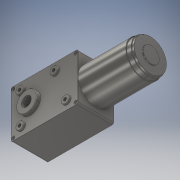
# Autodesk Inventor part: TS-58GZ868D
Saved by Autodesk Inventor 2018 (Build 220112000, 112)
## iProperties
Created: 2018-04-10
Part Number: TS-58GZ868D
Material: Steel, Cast
Document SubType Name: Modeling
Designer: P136265
Density: 7.85 g/cm^3
Appearance: Semi-Polished
Author: P136265
Autodesk Inventor part; units mm, degrees
ref_plane "YZ Plane" through (0, 0, 0) normal (1, 0, 0) x (0, 1, 0)
ref_plane "XZ Plane" through (0, 0, 0) normal (0, 1, 0) x (-1, 0, 0)
ref_plane "XY Plane" through (0, 0, 0) normal (0, 0, 1) x (1, 0, 0)
sketch "Sketch1" plane through (0, 0, 0) normal (0, 1, 0) x (-1, 0, 0)
  line L0 (-39.25, 29) -> (39.25, 29)
  line L1 (41.25, 27) -> (41.25, -27)
  line L2 (39.25, -29) -> (-39.25, -29)
  line L3 (-41.25, -27) -> (-41.25, 27)
  line L4 (-41.25, 29) -> (41.25, -29) construction
  line L5 (41.25, 29) -> (-41.25, -29) construction
  arc A0 (41.25, 27) -> (39.25, 29) centre (39.25, 27) ccw
  arc A1 (-39.25, 29) -> (-41.25, 27) centre (-39.25, 27) ccw
  arc A2 (-41.25, -27) -> (-39.25, -29) centre (-39.25, -27) ccw
  arc A3 (39.25, -29) -> (41.25, -27) centre (39.25, -27) ccw
  point P0 (0, 0)
  dimension "d0" = 82.5
  dimension "d1" = 58
  dimension "d2" = 2
  constraints: 12 end point, 8 point on circle, 8 point on line, 8 tangent, 4 centre point, 3 equal radius, 2 midpoint, 2 parallel, 1 horizontal, 1 perpendicular
  measures "d0" distance of L4.end L5.end
  measures "d1" distance of L5.start L4.end
  measures "d2" radius of A0
extrude "Extrusion1" add sketch "Sketch1" along normal mid plane 44
sketch "Sketch2" plane through (0, 22, 0) normal (0, 1, 0) x (1, 0, 0)
  line L0 (-41.25, 27) -> (-41.25, -27) construction
  arc A0 (-41.25, -27) -> (-39.25, -29) centre (-39.25, -27) ccw construction
  line L1 (-39.25, -29) -> (39.25, -29) construction
  arc A1 (39.25, -29) -> (41.25, -27) centre (39.25, -27) ccw construction
  line L2 (41.25, -27) -> (41.25, 27) construction
  arc A2 (41.25, 27) -> (39.25, 29) centre (39.25, 27) ccw construction
  line L3 (39.25, 29) -> (-39.25, 29) construction
  arc A3 (-39.25, 29) -> (-41.25, 27) centre (-39.25, 27) ccw construction
  line L4 (39.25, -29) -> (-39.25, -29) construction
  line L5 (28.25, -29) -> (28.25, 29) construction
  line L6 (-39.25, 29) -> (39.25, 29) construction
  line L7 (17.25, -29) -> (17.25, 29) construction
  circle A4 centre (17.25, 0) radius 12.5
  point P0 (0, 0)
  dimension "d5" = 13
  dimension "d7" = 11
  dimension "d8" = 25
  constraints: 4 end point, 4 point on line, 2 perpendicular, 1 centre point, 1 midpoint
  measures "d5" distance between parallel lines of L2 L5
  measures "d7" distance between parallel lines of L5 L7
  measures "d8" diameter of A4
extrude "Extrusion2" add sketch "Sketch2" along normal blind 5
sketch "Sketch3" plane through (0, 22, 0) normal (0, 1, 0) x (1, 0, 0)
  circle A0 centre (17.25, 0) radius 12.5 construction
  line L0 (-41.25, 27) -> (-41.25, -27) construction
  arc A1 (-41.25, -27) -> (-39.25, -29) centre (-39.25, -27) ccw construction
  line L1 (-39.25, -29) -> (39.25, -29) construction
  arc A2 (39.25, -29) -> (41.25, -27) centre (39.25, -27) ccw construction
  line L2 (41.25, -27) -> (41.25, 27) construction
  arc A3 (41.25, 27) -> (39.25, 29) centre (39.25, 27) ccw construction
  line L3 (39.25, 29) -> (-39.25, 29) construction
  arc A4 (-39.25, 29) -> (-41.25, 27) centre (-39.25, 27) ccw construction
  line L4 (28.25, -29) -> (28.25, 29) construction
  circle A5 centre (28.25, -19) radius 5
  circle A6 centre (28.25, 19) radius 5
  line L5 (28.25, 0) -> (17.25, 0) construction
  line L6 (-39.25, -29) -> (39.25, -29) construction
  line L7 (17.25, -29) -> (17.25, 29) construction
  line L8 (-13.75, -29) -> (-13.75, 29) construction
  line L9 (-27.75, -29) -> (-27.75, 29) construction
  circle A7 centre (-13.75, -19) radius 5
  circle A8 centre (-27.75, 19) radius 5
  line L10 (17.25, 0) -> (-27.75, 0) construction
  point P0 (0, 0)
  dimension "d11" = 13
  dimension "d12" = 10
  dimension "d13" = 10
  dimension "d14" = 38
  dimension "d15" = 19
  dimension "d19" = 31
  dimension "d20" = 45
  dimension "d21" = 10
  dimension "d22" = 10
  dimension "d23" = 19
  dimension "d24" = 19
  constraints: 12 end point, 12 point on line, 4 centre point, 4 perpendicular, 3 midpoint, 1 horizontal
  measures "d11" distance between parallel lines of L2 L4
  measures "d12" diameter of A5
  measures "d13" diameter of A6
  measures "d14" distance of A6.centre A5.centre
  measures "d15" distance of L5.start A5.centre
  measures "d19" distance from line of L5.end L8
  measures "d20" distance between parallel lines of L9 L7
  measures "d21" diameter of A7
  measures "d22" diameter of A8
  measures "d23" distance from line of L10 A8.centre
  measures "d24" distance from line of L10 A7.centre
extrude "Extrusion3" add sketch "Sketch3" along normal blind 2.5
fillet "Fillet1" radius 0.5 5 edges at (-18.75, 24.5, 19) (-32.75, 24.5, -19) (23.25, 24.5, 19) (23.25, 24.5, -19) (4.75, 27, 0)
mirror "Mirror1" about plane through (0, 0, 0) normal (0, 1, 0) of "Extrusion3", "Extrusion2", "Fillet1"
sketch "Sketch6" plane through (-13.75, 24.5, 19) normal (0, 1, 0) x (1, 0, 0)
  circle A0 centre (0, 0) radius 4.5 construction
  circle A1 centre (-14, 38) radius 4.5 construction
  circle A2 centre (42, 38) radius 4.5 construction
  circle A3 centre (42, 0) radius 4.5 construction
  point P0 (13.75, 19)
hole "Hole1" at (-13.75, 24.5, 19) at (-27.75, 24.5, -19) at (28.25, 24.5, -19) at (28.25, 24.5, 19) direction (0, -1, 0) diameter 4 end through all
thread "Thread1" size "M4x0.7" class "6H" standard "ANSI Metric M Profile" full length
thread "Thread2" size "M4x0.7" class "6H" standard "ANSI Metric M Profile" full length
thread "Thread3" size "M4x0.7" class "6H" standard "ANSI Metric M Profile" full length
thread "Thread4" size "M4x0.7" class "6H" standard "ANSI Metric M Profile" full length
sketch "Sketch7" plane through (-41.25, -22, 27) normal (-1, 0, 0) x (0, 0, 1)
  circle A0 centre (-27, 22) radius 22
  dimension "d51" = 44
  constraints: 1 centre point, 1 coincident
  measures "d51" diameter of A0
extrude "Extrusion6" add sketch "Sketch7" along normal blind 59
sketch "Sketch8" plane through (-100.25, 0, 0) normal (-1, 0, 0) x (0, 0, 1)
  circle A0 centre (0, 0) radius 21
  dimension "d54" = 42
  constraints: 1 centre point, 1 coincident
  measures "d54" diameter of A0
extrude "Extrusion7" add sketch "Sketch8" along normal blind 5.5
sketch "Sketch9" plane through (-105.75, 0, 0) normal (-1, 0, 0) x (0, 0, 1)
  circle A0 centre (0, 0) radius 20
  dimension "d57" = 40
  constraints: 1 centre point, 1 coincident
  measures "d57" diameter of A0
extrude "Extrusion8" add sketch "Sketch9" along normal blind 2.5
sketch "Sketch10" plane through (-108.25, 0, 0) normal (-1, 0, 0) x (0, 0, 1)
  circle A0 centre (0, 0) radius 10
  dimension "d60" = 20
  constraints: 1 centre point, 1 coincident
  measures "d60" diameter of A0
extrude "Extrusion9" add sketch "Sketch10" along normal blind 1
sketch "Sketch12" plane through (17.25, 27, 0) normal (0, 1, 0) x (1, 0, 0)
  circle A0 centre (0, 0) radius 12 construction
  circle A1 centre (0, 0) radius 6 construction
  point P0 (-17.25, 0)
  dimension "d99" = 12
  constraints: 1 centre point, 1 coincident
  measures "d99" diameter of A1
hole "Hole3" at (17.25, 27, 0) direction (0, -1, 0) diameter 12 end through all
fillet "Fillet2" radius 0.1 24 edges at (-109.25, 0, -10) (-108.25, 0, -20) (-105.75, 0, -21) (-100.25, 0, -22) (-40.6642, -22, 28.4142) (0, -22, 29) (40.6642, -22, 28.4142) (41.25, -22, 0) (40.6642, -22, -28.4142) (0, -22, -29) (-40.6642, -22, -28.4142) (-41.25, -22, -13.5) (-41.25, -22, 13.5) (-40.6642, 22, 28.4142) (0, 22, 29) (40.6642, 22, 28.4142) (41.25, 22, 0) (40.6642, 22, -28.4142) (0, 22, -29) (-40.6642, 22, -28.4142) (-41.25, 22, -13.5) (-41.25, 22, 13.5) (17.25, 27, -6) (17.25, -27, -6)
sketch "Sketch11" plane through (0, 22, 0) normal (0, 1, 0) x (1, 0, 0)
  line L0 (-41.15, -27) -> (-41.15, -2.0952) construction
  arc A0 (-41.15, -27) -> (-39.25, -28.9) centre (-39.25, -27) ccw construction
  line L1 (39.25, -28.9) -> (-39.25, -28.9) construction
  arc A1 (39.25, -28.9) -> (41.15, -27) centre (39.25, -27) ccw construction
  line L2 (41.15, 27) -> (41.15, -27) construction
  arc A2 (41.15, 27) -> (39.25, 28.9) centre (39.25, 27) ccw construction
  line L3 (-39.25, 28.9) -> (39.25, 28.9) construction
  arc A3 (-39.25, 28.9) -> (-41.15, 27) centre (-39.25, 27) ccw construction
  line L4 (-41.15, 2.0952) -> (-41.15, 27) construction
  circle A4 centre (-13.75, -19) radius 5 construction
  circle A5 centre (28.25, -19) radius 5 construction
  circle A6 centre (28.25, 19) radius 5 construction
  circle A7 centre (-27.75, 19) radius 5 construction
  circle A8 centre (17.25, 0) radius 12.5 construction
  circle A9 centre (-38.25, -26) radius 2 construction
  circle A10 centre (-38.25, 26) radius 2 construction
  circle A11 centre (38.25, 26) radius 2 construction
  circle A12 centre (38.25, -26) radius 2 construction
  point P0 (0, 0)
  dimension "d52" = 59
  dimension "d64" = 4
  dimension "d65" = 1
  dimension "d66" = 1
  dimension "d67" = 4
  dimension "d68" = 1
  dimension "d69" = 1
  dimension "d70" = 4
  dimension "d71" = 1
  dimension "d72" = 1
  dimension "d73" = 4
  dimension "d74" = 1
  dimension "d75" = 1
  constraints: 4 centre point, 2 other
  measures "d64" diameter of A9
  measures "d65" horizontal distance of A0.centre A9.centre
  measures "d66" horizontal distance of A0.centre A9.centre
  measures "d67" diameter of A10
  measures "d68" horizontal distance of A3.centre A10.centre
  measures "d69" horizontal distance of A3.centre A10.centre
  measures "d70" diameter of A11
  measures "d71" horizontal distance of A2.centre A11.centre
  measures "d72" horizontal distance of A2.centre A11.centre
  measures "d73" diameter of A12
  measures "d74" horizontal distance of A1.centre A12.centre
  measures "d75" horizontal distance of A1.centre A12.centre
hole "Hole2" at (38.25, 22, 26) at (38.25, 22, -26) at (-38.25, 22, -26) at (-38.25, 22, 26) direction (0, -1, 0) diameter 2 depth 8 tip angle 118 counterbore diameter 4 counterbore depth 2
thread "Thread5" size "M2x0.4" class "6H" standard "ANSI Metric M Profile" full length
thread "Thread6" size "M2x0.4" class "6H" standard "ANSI Metric M Profile" full length
thread "Thread7" size "M2x0.4" class "6H" standard "ANSI Metric M Profile" full length
thread "Thread8" size "M2x0.4" class "6H" standard "ANSI Metric M Profile" full length
mirror "Mirror2" about plane through (0, 0, 0) normal (0, 1, 0) of "Hole2"
thread "Thread9" size "M2x0.4" class "6H" standard "ANSI Metric M Profile" full length
thread "Thread10" size "M2x0.4" class "6H" standard "ANSI Metric M Profile" full length
thread "Thread11" size "M2x0.4" class "6H" standard "ANSI Metric M Profile" full length
thread "Thread12" size "M2x0.4" class "6H" standard "ANSI Metric M Profile" full length
body "Solid1"
